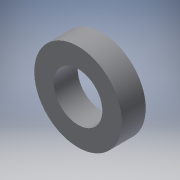
# Autodesk Inventor part: Distance_lin
Saved by Autodesk Inventor 2019.3 (Build 233278000, 278)
## iProperties
Created: 2020-09-08
Part Number: Distance_lin
Material: Generisch
Document SubType Name: Modeling
Designer: Nicolas Frick
Density: 1 g/cm^3
Appearance: Vorgabe
Author: Nicolas Frick
Autodesk Inventor part; units mm, degrees
ref_plane "YZ Plane" through (0, 0, 0) normal (1, 0, 0) x (0, 1, 0)
ref_plane "XZ Plane" through (0, 0, 0) normal (0, 1, 0) x (-1, 0, 0)
ref_plane "XY Plane" through (0, 0, 0) normal (0, 0, 1) x (1, 0, 0)
sketch "Skizze1" plane through (0, 0, 0) normal (0, 0, 1) x (1, 0, 0)
  arc A0 (-9.5959, 5.5794) -> (9.5959, -5.5794) centre (0, 0) ccw construction
  circle A1 centre (0, 0) radius 6 construction
  circle A2 centre (0, 0) radius 11 construction
  circle A3 centre (0, 0) radius 6.1
  circle A4 centre (0, 0) radius 11
  point P0 (0, 0)
  dimension "d0" = 12.2
  constraints: 2 centre point, 2 coincident, 1 concentric
  measures "d0" diameter of A3
extrude "Extrusion1" add sketch "Skizze1" along normal blind 6
